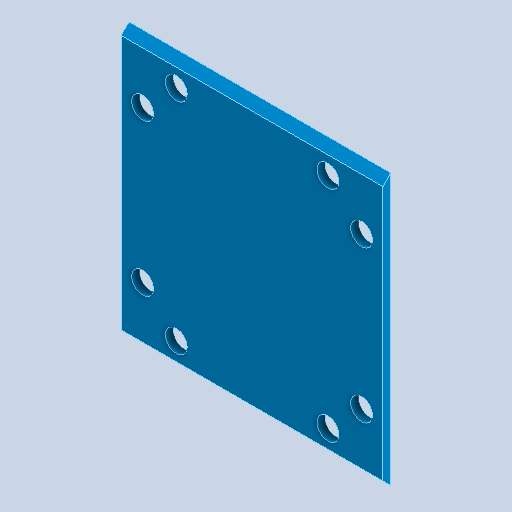
# Autodesk Inventor part: Panel Top 1x1
Saved by Autodesk Inventor 2023.1 (Build 271208000, 208)
## iProperties
Created: 2022-08-10
Part Number: Panel Top 1x1
Material: Generic
Document SubType Name: Modeling
Designer: xSibe
Density: 1 g/cm^3
Appearance: Plastic Teal
Author: xSibe
Autodesk Inventor part; units mm, degrees
ref_plane "YZ Plane" through (0, 0, 0) normal (1, 0, 0) x (0, 1, 0)
ref_plane "XZ Plane" through (0, 0, 0) normal (0, 1, 0) x (-1, 0, 0)
sketch "Sketch1" plane through (0, 0, 0) normal (0, 0, 1) x (1, 0, 0)
  circle A0 centre (-21.9, -21.9) radius 1.875 projected
  circle A1 centre (21.9, 21.9) radius 1.875 projected
  circle A2 centre (21.9, -21.9) radius 1.875 projected
  circle A3 centre (-21.9, 21.9) radius 1.875 projected
  circle A4 centre (14.4, 20.8) radius 2.0734 projected
  circle A5 centre (-14.4, -20.8) radius 2.0734 projected
  circle A6 centre (14.4, -20.8) radius 2.0734 projected
  circle A7 centre (20.8, -14.4) radius 2.0734 projected
  line L0 (-17.05, 17.05) -> (-17.05, -17.05) projected
  line L1 (17.05, 17.05) -> (-17.05, 17.05) projected
  line L2 (17.05, -17.05) -> (17.05, 17.05) projected
  line L3 (-17.05, -17.05) -> (17.05, -17.05) projected
  circle A8 centre (20.8, 14.4) radius 2.0734 projected
  circle A9 centre (-14.4, 20.8) radius 2.0734 projected
  circle A10 centre (-20.8, -14.4) radius 2.0734 projected
  circle A11 centre (-20.8, 14.4) radius 2.0734 projected
  line L4 (-22.9, 24.875) -> (22.9, 24.875) projected
  arc A12 (-22.9, 24.875) -> (-24.875, 22.9) centre (-22.9, 22.9) ccw projected
  line L5 (-24.875, -22.9) -> (-24.875, 22.9) projected
  arc A13 (-24.875, -22.9) -> (-22.9, -24.875) centre (-22.9, -22.9) ccw projected
  line L6 (22.9, -24.875) -> (-22.9, -24.875) projected
  arc A14 (22.9, -24.875) -> (24.875, -22.9) centre (22.9, -22.9) ccw projected
  line L7 (24.875, 22.9) -> (24.875, -22.9) projected
  arc A15 (24.875, 22.9) -> (22.9, 24.875) centre (22.9, 22.9) ccw projected
  point P0 (0, 0)
ref_plane "Work Plane1" through (-24.15, -24.15, 49.8) normal (0, 0, 1) x (1, 0, 0)
extrude "Extrusion1" add sketch "Sketch1" along normal blind 1.5 from surface at 49.8 contours A0 | A1 | A2 | A3 | L1 L2 L3 L0 | L4 A15 L7 A14 L6 A13 L5 A12
sketch "Sketch2" plane through (-22.9, -24.875, 51.3) normal (0, 0, 1) x (1, 0, 0)
  arc A0 (-1.975, 1.975) -> (0, 0) centre (0, 1.975) ccw projected
  line L0 (45.8, 0) -> (0, 0) projected
  arc A1 (45.8, 0) -> (47.775, 1.975) centre (45.8, 1.975) ccw projected
  line L1 (47.775, 47.775) -> (47.775, 1.975) projected
  arc A2 (47.775, 47.775) -> (45.8, 49.75) centre (45.8, 47.775) ccw projected
  line L2 (0, 49.75) -> (45.8, 49.75) projected
  arc A3 (0, 49.75) -> (-1.975, 47.775) centre (0, 47.775) ccw projected
  line L3 (-1.975, 1.975) -> (-1.975, 47.775) projected
  circle A4 centre (2.1, 39.275) radius 2.0734 projected
  circle A5 centre (2.1, 10.475) radius 2.0734 projected
  circle A6 centre (8.5, 45.675) radius 2.0734 projected
  circle A7 centre (43.7, 39.275) radius 2.0734 projected
  circle A8 centre (43.7, 10.475) radius 2.0734 projected
  circle A9 centre (37.3, 4.075) radius 2.0734 projected
  circle A10 centre (8.5, 4.075) radius 2.0734 projected
  circle A11 centre (37.3, 45.675) radius 2.0734 projected
  arc A12 (48.625, 47.775) -> (45.8, 50.6) centre (45.8, 47.775) ccw
  line L4 (48.625, 47.775) -> (48.625, 1.975)
  arc A13 (45.8, -0.85) -> (48.625, 1.975) centre (45.8, 1.975) ccw
  line L5 (45.8, -0.85) -> (0, -0.85)
  arc A14 (-2.825, 1.975) -> (0, -0.85) centre (0, 1.975) ccw
  line L6 (-2.825, 1.975) -> (-2.825, 47.775)
  arc A15 (0, 50.6) -> (-2.825, 47.775) centre (0, 47.775) ccw
  line L7 (0, 50.6) -> (45.8, 50.6)
  line L8 (47.775, 1.975) -> (45.8, 1.975)
  line L9 (45.8, 1.975) -> (45.8, -0.85)
  line L10 (45.8, -0.85) -> (47.775, -0.85)
  line L11 (47.775, -0.85) -> (47.775, 1.975)
  line L12 (-1.975, 1.975) -> (0, 1.975)
  line L13 (0, 1.975) -> (0, -0.85)
  line L14 (0, -0.85) -> (-1.975, -0.85)
  line L15 (-1.975, -0.85) -> (-1.975, 1.975)
  line L16 (-1.975, 47.775) -> (0, 47.775)
  line L17 (0, 47.775) -> (0, 50.6)
  line L18 (0, 50.6) -> (-1.975, 50.6)
  line L19 (-1.975, 50.6) -> (-1.975, 47.775)
  line L20 (47.775, 47.775) -> (45.8, 47.775)
  line L21 (45.8, 47.775) -> (45.8, 50.6)
  line L22 (45.8, 50.6) -> (47.775, 50.6)
  line L23 (47.775, 50.6) -> (47.775, 47.775)
  point P0 (22.9, 24.875)
  dimension "d2" = 0.85
  constraints: 40 end point, 8 parallel, 8 point on circle, 4 centre point, 4 horizontal, 4 perpendicular, 7 other
  measures "d2" distance between parallel lines of L2 L7
extrude "Extrusion2" add sketch "Sketch2" against normal blind 1.5 contours A0 L13 A14 L15 | L0 L9 L5 L13 | L19 A15 L17 A3 | A14 L14 L15 | A1 L11 A13 L9 | L17 L7 L21 L2 | L19 L18 A15 | A13 L11 L10 | L21 A12 L23 A2 | L22 L23 A12
chamfer "Chamfer1" distance 1.5 angle 45 2 edges at (0, 25.725, 51.3) (0, -25.725, 51.3)
body "Solid1"
